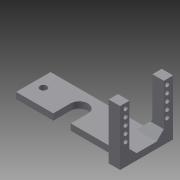
# Autodesk Inventor part: Servo-Groove-Mount-J-Head
Saved by Autodesk Inventor 2013 (Build 170138000, 138)
## iProperties
Created: 2013-11-15
Part Number: Servo-Groove-Mount-J-Head
Material: Generic
Document SubType Name: Modeling
Designer: Enlightx
Density: 1 g/cm^3
Author: Enlightx
Autodesk Inventor part; units mm, degrees
ref_plane "YZ Plane" through (0, 0, 0) normal (1, 0, 0) x (0, 1, 0)
ref_plane "XZ Plane" through (0, 0, 0) normal (0, 1, 0) x (-1, 0, 0)
ref_plane "XY Plane" through (0, 0, 0) normal (0, 0, 1) x (1, 0, 0)
sketch "Sketch1" plane through (0, 0, 0) normal (0, 0, 1) x (1, 0, 0)
  line L0 (-39.5, 12) -> (39.5, 12)
  line L1 (39.5, 12) -> (39.5, -12)
  line L2 (39.5, -12) -> (-39.5, -12)
  line L3 (-39.5, -12) -> (-39.5, 12)
  line L4 (-39.5, 12) -> (39.5, -12) construction
  line L5 (39.5, 12) -> (-39.5, -12) construction
  point P0 (0, 0)
  dimension "d0" = 79
  dimension "d1" = 24
  constraints: 12 end point, 2 midpoint, 2 parallel, 1 horizontal, 1 perpendicular
  measures "d0" distance of L1.end L2.end
  measures "d1" distance of L0.end L1.end
extrude "Extrusion1" add sketch "Sketch1" along normal blind 4.4
sketch "Sketch3" plane through (0, 0, 0) normal (0, 0, -1) x (-1, 0, 0)
  line L0 (-39.5, 12) -> (-31.5, 12)
  line L1 (-31.5, 12) -> (-31.5, 18.5)
  line L2 (-31.5, 18.5) -> (-39.5, 18.5)
  line L3 (-39.5, 18.5) -> (-39.5, 12)
  line L4 (-39.5, -12) -> (-31.5, -12)
  line L5 (-31.5, -12) -> (-31.5, -18.5)
  line L6 (-31.5, -18.5) -> (-39.5, -18.5)
  line L7 (-39.5, -18.5) -> (-39.5, -12)
  point P0 (0, 0)
  dimension "d8" = 8
  dimension "d9" = 6.5
  dimension "d10" = 6.5
  constraints: 16 end point, 4 parallel, 2 horizontal, 2 perpendicular
  measures "d8" distance of L2.end L1.end
  measures "d9" distance of L1.end L0.end
  measures "d10" distance of L4.end L5.end
extrude "Extrusion2" add sketch "Sketch3" against normal blind 38.6
chamfer "Chamfer1" distance 6.5 angle 45 2 edges at (31.5, -12, 2.2) (31.5, 12, 2.2)
sketch "Sketch5" plane through (0, 0, 0) normal (0, 0, -1) x (-1, 0, 0)
  line L0 (-25, -12) -> (39.5, -12) projected
  line L1 (39.5, 12) -> (-24.5, 12) construction
  line L2 (-24.5, 12) -> (-24.5, -12) construction
  line L3 (-24.5, -12) -> (39.5, -12) construction
  line L4 (39.5, -12) -> (39.5, 12) construction
  line L5 (-24.5, 12) -> (39.5, -12) construction
  line L6 (39.5, 12) -> (-24.5, -12) construction
  circle A0 centre (7.5, 0) radius 6.1
  line L7 (-17.5, 3) -> (32.5, 3) construction
  line L8 (32.5, 3) -> (32.5, -3) construction
  line L9 (32.5, -3) -> (-17.5, -3) construction
  line L10 (-17.5, -3) -> (-17.5, 3) construction
  line L11 (-17.5, 3) -> (32.5, -3) construction
  line L12 (32.5, 3) -> (-17.5, -3) construction
  circle A1 centre (-17.5, 0) radius 2.4
  circle A2 centre (32.5, 0) radius 2.4
  line L13 (1.4, 0) -> (1.4, -12)
  line L14 (13.6, 0) -> (13.6, -12)
  line L15 (13.6, -12) -> (1.4, -12)
  point P0 (0, 0)
  dimension "d29" = 64
  dimension "d30" = 12.2
  dimension "d31" = 50
  dimension "d32" = 4.8
  dimension "d33" = 4.8
  constraints: 30 end point, 5 midpoint, 4 parallel, 4 perpendicular, 3 centre point, 3 point on line, 2 horizontal, 2 point on circle, 2 tangent, 1 collinear
  measures "d29" distance of L3.end L2.end
  measures "d30" diameter of A0
  measures "d31" distance of L8.end L9.end
  measures "d32" diameter of A1
  measures "d33" diameter of A2
extrude "Extrusion4" cut sketch "Sketch5" against normal blind 5.6
sketch "Sketch6" plane through (39.5, -18.5, 0) normal (1, 0, 0) x (0, 0, -1)
  line L0 (-38.6, 6.5) -> (-5.6, 6.5) construction
  line L1 (-5.6, 6.5) -> (-5.6, 1.5) construction
  line L2 (-5.6, 1.5) -> (-38.6, 1.5) construction
  line L3 (-38.6, 1.5) -> (-38.6, 6.5) construction
  line L4 (-38.6, 30.5) -> (-5.6, 30.5) construction
  line L5 (-5.6, 30.5) -> (-5.6, 35.5) construction
  line L6 (-5.6, 35.5) -> (-38.6, 35.5) construction
  line L7 (-38.6, 35.5) -> (-38.6, 30.5) construction
  line L8 (-38.6, 4) -> (-5.6, 4) construction
  line L9 (-38.6, 33) -> (-5.6, 33) construction
  line L10 (-38.6, 1.5) -> (-37.6, 1.5) construction
  line L11 (-37.6, 1.5) -> (-37.6, 6.5) construction
  line L12 (-37.6, 6.5) -> (-38.6, 6.5) construction
  line L13 (-38.6, 6.5) -> (-38.6, 1.5) construction
  line L14 (-37.6, 1.5) -> (-32.6, 1.5) construction
  line L15 (-32.6, 1.5) -> (-32.6, 6.5) construction
  line L16 (-32.6, 6.5) -> (-37.6, 6.5) construction
  line L17 (-37.6, 6.5) -> (-37.6, 1.5) construction
  line L18 (-38.6, 30.5) -> (-37.6, 30.5) construction
  line L19 (-37.6, 30.5) -> (-37.6, 35.5) construction
  line L20 (-37.6, 35.5) -> (-38.6, 35.5) construction
  line L21 (-38.6, 35.5) -> (-38.6, 30.5) construction
  line L22 (-37.6, 30.5) -> (-32.6, 30.5) construction
  line L23 (-32.6, 30.5) -> (-32.6, 35.5) construction
  line L24 (-32.6, 35.5) -> (-37.6, 35.5) construction
  line L25 (-37.6, 35.5) -> (-37.6, 30.5) construction
  line L26 (-37.6, 1.5) -> (-32.6, 6.5) construction
  line L27 (-37.6, 6.5) -> (-32.6, 1.5) construction
  line L28 (-37.6, 30.5) -> (-32.6, 35.5) construction
  line L29 (-37.6, 35.5) -> (-32.6, 30.5) construction
  line L30 (-38.6, 35.5) -> (-37.6, 35.5) construction
  line L31 (-37.6, 35.5) -> (-37.6, 30.5) construction
  line L32 (-37.6, 30.5) -> (-38.6, 30.5) construction
  line L33 (-38.6, 30.5) -> (-38.6, 35.5) construction
  line L34 (-4.4, 30.5) -> (-38.6, 30.5) projected
  line L35 (-32.6, 35.5) -> (-27.6, 35.5) construction
  line L36 (-27.6, 35.5) -> (-27.6, 30.5) construction
  line L37 (-27.6, 30.5) -> (-32.6, 30.5) construction
  line L38 (-32.6, 30.5) -> (-32.6, 35.5) construction
  line L39 (-27.6, 35.5) -> (-22.6, 35.5) construction
  line L40 (-22.6, 35.5) -> (-22.6, 30.5) construction
  line L41 (-22.6, 30.5) -> (-27.6, 30.5) construction
  line L42 (-27.6, 30.5) -> (-27.6, 35.5) construction
  line L43 (-32.6, 6.5) -> (-27.6, 6.5) construction
  line L44 (-27.6, 6.5) -> (-27.6, 1.5) construction
  line L45 (-27.6, 1.5) -> (-32.6, 1.5) construction
  line L46 (-32.6, 1.5) -> (-32.6, 6.5) construction
  line L47 (-27.6, 6.5) -> (-22.6, 6.5) construction
  line L48 (-22.6, 6.5) -> (-22.6, 1.5) construction
  line L49 (-22.6, 1.5) -> (-27.6, 1.5) construction
  line L50 (-27.6, 1.5) -> (-27.6, 6.5) construction
  line L51 (-22.6, 35.5) -> (-17.6, 35.5) construction
  line L52 (-17.6, 35.5) -> (-17.6, 30.5) construction
  line L53 (-17.6, 30.5) -> (-22.6, 30.5) construction
  line L54 (-22.6, 30.5) -> (-22.6, 35.5) construction
  line L55 (-22.6, 6.5) -> (-17.6, 6.5) construction
  line L56 (-17.6, 6.5) -> (-17.6, 1.5) construction
  line L57 (-17.6, 1.5) -> (-22.6, 1.5) construction
  line L58 (-22.6, 1.5) -> (-22.6, 6.5) construction
  line L59 (-17.6, 35.5) -> (-12.6, 35.5) construction
  line L60 (-12.6, 35.5) -> (-12.6, 30.5) construction
  line L61 (-12.6, 30.5) -> (-17.6, 30.5) construction
  line L62 (-17.6, 30.5) -> (-17.6, 35.5) construction
  line L63 (-17.6, 6.5) -> (-12.6, 6.5) construction
  line L64 (-12.6, 6.5) -> (-12.6, 1.5) construction
  line L65 (-12.6, 1.5) -> (-17.6, 1.5) construction
  line L66 (-17.6, 1.5) -> (-17.6, 6.5) construction
  line L67 (-32.6, 35.5) -> (-27.6, 30.5) construction
  line L68 (-27.6, 35.5) -> (-32.6, 30.5) construction
  line L69 (-27.6, 35.5) -> (-22.6, 30.5) construction
  line L70 (-27.6, 30.5) -> (-22.6, 35.5) construction
  line L71 (-22.6, 30.5) -> (-17.6, 35.5) construction
  line L72 (-22.6, 35.5) -> (-17.6, 30.5) construction
  line L73 (-17.6, 35.5) -> (-12.6, 30.5) construction
  line L74 (-12.6, 35.5) -> (-17.6, 30.5) construction
  line L75 (-17.6, 6.5) -> (-12.6, 1.5) construction
  line L76 (-12.6, 6.5) -> (-17.6, 1.5) construction
  line L77 (-22.6, 6.5) -> (-17.6, 1.5) construction
  line L78 (-17.6, 6.5) -> (-22.6, 1.5) construction
  line L79 (-27.6, 6.5) -> (-22.6, 1.5) construction
  line L80 (-22.6, 6.5) -> (-27.6, 1.5) construction
  line L81 (-32.6, 6.5) -> (-27.6, 1.5) construction
  line L82 (-27.6, 6.5) -> (-32.6, 1.5) construction
  point P0 (0, 18.5)
  point P1 (-35.1, 4)
  point P2 (-35.1, 33)
  point P3 (-30.1, 33)
  point P4 (-25.1, 33)
  point P5 (-20.1, 33)
  point P6 (-15.1, 33)
  point P7 (-15.1, 4)
  point P8 (-20.1, 4)
  point P9 (-25.1, 4)
  point P10 (-30.1, 4)
  dimension "d42" = 5
  dimension "d43" = 5
  dimension "d44" = 1
  dimension "d45" = 5
  dimension "d46" = 5
  dimension "d54" = 33
  dimension "d55" = 1
  dimension "d59" = 5
  dimension "d60" = 5
  dimension "d61" = 5
  dimension "d62" = 5
  constraints: 164 end point, 32 parallel, 24 perpendicular, 21 point on line, 15 horizontal, 15 midpoint
  measures "d42" distance of L0.end L1.end
  measures "d43" distance of L5.end L4.end
  measures "d44" distance of L12.end L11.end
  measures "d45" distance of L16.end L15.end
  measures "d46" distance of L24.end L23.end
  measures "d54" distance of L4.start L4.end
  measures "d55" distance of L18.end L32.end
  measures "d59" distance of L36.end L37.end
  measures "d60" distance of L40.end L41.end
  measures "d61" distance of L52.end L53.end
  measures "d62" distance of L60.end L61.end
hole "Hole2" at (39.5, -14.5, 35.1) at (39.5, 14.5, 35.1) at (39.5, 14.5, 30.1) at (39.5, 14.5, 25.1) at (39.5, 14.5, 20.1) at (39.5, 14.5, 15.1) at (39.5, -14.5, 15.1) at (39.5, -14.5, 20.1) at (39.5, -14.5, 25.1) at (39.5, -14.5, 30.1) direction (-1, 0, 0) diameter 3 end through all
chamfer "Chamfer2" distance 6.4 angle 45 2 edges at (31.5, 15.25, 4.4) (31.5, -15.25, 4.4)
chamfer "Chamfer3" distance 5 angle 45 2 edges at (35.5, 12, 4.4) (35.5, -12, 4.4)
body "Solid1"
